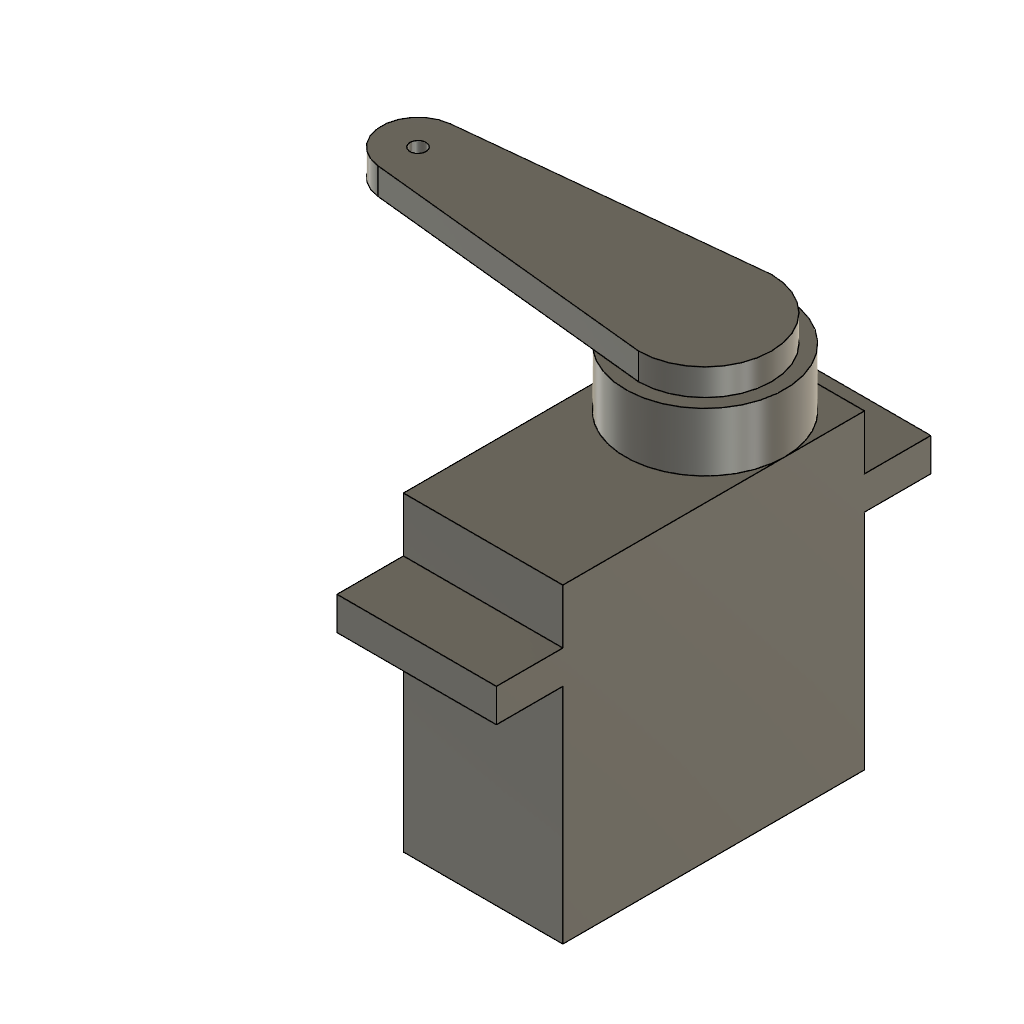
v1 (Autodesk Fusion 360 archive; units mm, degrees)
design "servo"
Autodesk Fusion 360 part; units mm, degrees
sketch "Sketch1" plane through (0, 0, 0) normal (0, 0, 1) x (1, 0, 0)
  line L0 (6, -11.35) -> (-6, -11.35)
  line L1 (-6, -11.35) -> (-6, 11.35)
  line L2 (-6, 11.35) -> (6, 11.35)
  line L3 (6, 11.35) -> (6, -11.35)
  line L4 (6, -11.35) -> (-6, 11.35) construction
  line L5 (-6, -11.35) -> (6, 11.35) construction
  dimension "d1" = 12
  dimension "d2" = 22.7
  constraint horizontal L0
  constraint perpendicular L0 L1
  constraint parallel L0 L2
  constraint parallel L1 L3
  constraint coincident L4 origin
  constraint coincident L5 origin
  measures "d1" distance of L1.end L2.end
  measures "d2" distance of L0.end L1.end
extrude "Extrude1" add sketch "Sketch1" along normal blind 16.8 makes body 1
sketch "Sketch2" plane through (0, 0, 16.8) normal (0, 0, 1) x (-1, 0, 0)
  line L0 (-6, -11.35) -> (6, -11.35)
  line L1 (6, -11.35) -> (6, 11.35)
  line L2 (6, 11.35) -> (-6, 11.35)
  line L3 (-6, 11.35) -> (-6, -11.35)
  line L4 (-6, 16.35) -> (6, 16.35)
  line L5 (6, 16.35) -> (6, -16.35)
  line L6 (6, -16.35) -> (-6, -16.35)
  line L7 (-6, -16.35) -> (-6, 16.35)
  line L8 (-6, 16.35) -> (6, -16.35) construction
  line L9 (6, 16.35) -> (-6, -16.35) construction
  dimension "d5" = 12
  dimension "d6" = 32.7
  constraint horizontal L4
  constraint perpendicular L4 L5
  constraint parallel L4 L6
  constraint parallel L5 L7
  constraint coincident L8 origin
  constraint coincident L9 origin
  measures "d5" distance of L5.end L6.end
  measures "d6" distance of L4.end L5.end
extrude "Extrude2" add sketch "Sketch2" along normal blind 2.5 separate body contours L0 L5 L6 L7 | L2 L4 L5 L7 makes body 2 at (2, -14.6833, 16.8) makes body 3 at (2, 13.0167, 16.8)
extrude "Extrude3" add 1 faces at (2, -3.7833, 16.8) along direction (0, 0, 1) blind 6.6 on bodies 1 bodies 1 2 3
sketch "Sketch3" plane through (0, 0, 23.4) normal (0, 0, 1) x (-1, 0, 0)
  line L0 (-6, -11.35) -> (6, -11.35)
  line L1 (6, -11.35) -> (6, 11.35)
  line L2 (6, 11.35) -> (-6, 11.35)
  line L3 (-6, 11.35) -> (-6, -11.35)
  circle A0 centre (0, -11.35) radius 6
  circle A1 centre (0, -5.35) radius 6
  constraint midpoint L0 A0.centre
  constraint coincident L0.end A0
  constraint coincident A0 A1.centre
  constraint coincident A0.centre A1
  constraint tangent L0 A1
extrude "Extrude4" add sketch "Sketch3" along normal blind 4.4 contours A0 A1 | A0 A1 bodies 1
sketch "Sketch4" plane through (0, 0, 27.8) normal (0, 0, 1) x (-1, 0, 0)
  circle A0 centre (0, -5.35) radius 6
  circle A1 centre (0, -5.35) radius 5
  line L0 (5, -5.35) -> (21, -5.35)
  circle A2 centre (21.6, -5.3517) radius 0.6
  circle A3 centre (21.6, -5.3517) radius 2.75
  line L1 (0, -10.35) -> (21.8829, -8.0871)
  line L2 (0, -0.35) -> (21.8833, -2.6163)
  dimension "d13" = 10
  dimension "d14" = 16
  dimension "d15" = 1.2
  dimension "d16" = 5.5
  constraint concentric A0 A1
  constraint coincident A1 L0.start
  constraint perpendicular A1 L0
  constraint coincident L0.end A2
  constraint concentric A2 A3
  constraint coincident A1 L1.start
  constraint coincident A3 L1.end
  constraint tangent A3 L1
  constraint coincident A1 L2.start
  constraint coincident A3 L2.end
  constraint tangent A3 L2
  measures "d13" diameter of A1
  measures "d14" distance of L0.start L0.end
  measures "d15" diameter of A2
  measures "d16" diameter of A3
extrude "Extrude5" add sketch "Sketch4" along normal blind 2 contours A0 A1 L0 L2 | A0 L0 A3 L1 | A0 A1 L0 L1 | A0 L0 A3 L2 | A1 L1 L2 | A3 bodies 1
